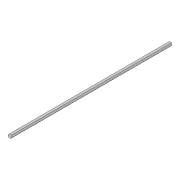
# Autodesk Inventor part: cross shaft
Saved by Autodesk Inventor 2018 (Build 220112000, 112)
## iProperties
Created: 2017-12-19
Part Number: cross shaft
Material: Generic
Document SubType Name: Modeling
Designer: dsayers
Density: 1 g/cm^3
Appearance: Default
Author: dsayers
Autodesk Inventor part; units mm, degrees
ref_plane "YZ Plane" through (0, 0, 0) normal (1, 0, 0) x (0, 1, 0)
ref_plane "XZ Plane" through (0, 0, 0) normal (0, 1, 0) x (-1, 0, 0)
ref_plane "XY Plane" through (0, 0, 0) normal (0, 0, 1) x (1, 0, 0)
sketch "Sketch1" plane through (0, 0, 0) normal (0, 0, 1) x (1, 0, 0)
  line L0 (1.9462, 2.1321) -> (2.8195, -0.6194)
  line L1 (2.8195, -0.6194) -> (0.8734, -2.7515)
  line L2 (0.8734, -2.7515) -> (-1.9462, -2.1321)
  line L3 (-1.9462, -2.1321) -> (-2.8195, 0.6194)
  line L4 (-2.8195, 0.6194) -> (-0.8734, 2.7515)
  line L5 (-0.8734, 2.7515) -> (1.9462, 2.1321)
  point P0 (0, 0)
  point P1 (0, 0)
  dimension "d0" = 5
  constraints: 12 end point, 1 coincident, 13 other
  measures "d0" distance between parallel lines of L2 L5
extrude "Extrusion1" add sketch "Sketch1" along normal blind 241.3
body "Solid1"
